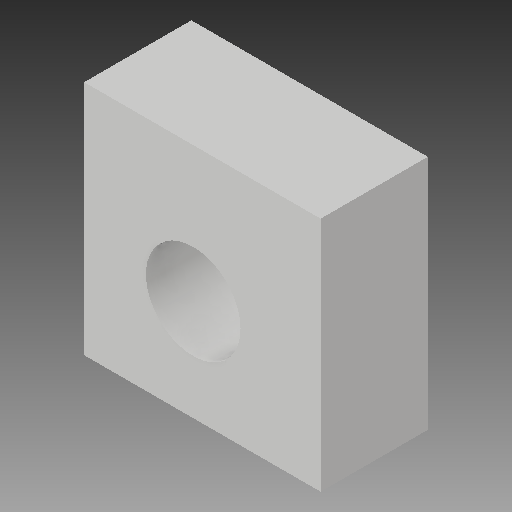
# Autodesk Inventor part: Fixer
Saved by Autodesk Inventor 2019 (Build 230136000, 136)
## iProperties
Created: 2021-11-07
Part Number: Fixer
Material: Generic
Document SubType Name: Modeling
Designer: Mohamed Teleb
Density: 1 g/cm^3
Appearance: Default
Author: Mohamed Teleb
Autodesk Inventor part; units mm, degrees
ref_plane "YZ Plane" through (0, 0, 0) normal (1, 0, 0) x (0, 1, 0)
ref_plane "XZ Plane" through (0, 0, 0) normal (0, 1, 0) x (-1, 0, 0)
ref_plane "XY Plane" through (0, 0, 0) normal (0, 0, 1) x (1, 0, 0)
sketch "Sketch1" plane through (0, 0, 0) normal (0, 0, 1) x (1, 0, 0)
  line L0 (-5.4538, 6.4099) -> (9.5462, 6.4099)
  line L1 (9.5462, 6.4099) -> (9.5462, -8.5901)
  line L2 (9.5462, -8.5901) -> (-5.4538, -8.5901)
  line L3 (-5.4538, -8.5901) -> (-5.4538, 6.4099)
  point P0 (0, 0)
  dimension "d0" = 15
  dimension "d1" = 15
  constraints: 8 end point, 2 parallel, 1 horizontal, 1 perpendicular
  measures "d0" distance of L1.end L2.end
  measures "d1" distance of L0.end L1.end
extrude "Extrusion1" add sketch "Sketch1" along normal blind 6.8
sketch "Sketch2" plane through (0, 0, 6.8) normal (0, 0, 1) x (1, 0, 0)
  circle A0 centre (1.4656, -2.1794) radius 3 projected
  circle A1 centre (1.4656, -2.1794) radius 3
  point P0 (0, 0)
  constraints: 1 centre point, 1 coincident, 1 concentric
extrude "Extrusion2" cut sketch "Sketch2" against normal blind 14
body "Solid1"
